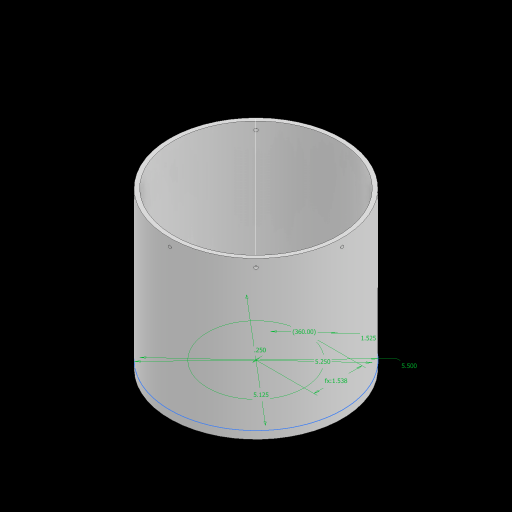
# Autodesk Inventor part: SC-1-01-Housing for Ice Holder
Saved by Autodesk Inventor 2023 (Build 270158000, 158)
## iProperties
Created: 2023-12-31
Part Number: SC-1-01-Housing for Ice Holder
Material: Generic
Document SubType Name: Modeling
Designer: annah
Density: 1 g/cm^3
Appearance: Default
Author: annah
Autodesk Inventor part; units mm, degrees
ref_plane "YZ Plane" through (0, 0, 0) normal (1, 0, 0) x (0, 1, 0)
ref_plane "XZ Plane" through (0, 0, 0) normal (0, 1, 0) x (-1, 0, 0)
sketch "Sketch1" plane through (0, 0, 0) normal (0, 1, 0) x (-1, 0, 0)
  circle A0 centre (0, 0) radius 66.675
  circle A1 centre (0, 0) radius 65.0875
  circle A2 centre (0, -39.0525) radius 19.3675
  circle A3 centre (39.0525, 0) radius 19.3675
  circle A4 centre (0, 39.0525) radius 19.3675
  circle A5 centre (-39.0525, 0) radius 19.3675
  circle A6 centre (0, 0) radius 3.175
  circle A7 centre (0, 0) radius 69.85
  dimension "d0" = 133.35
  dimension "d3" = 130.175
  dimension "d4" = 38.735
  dimension "d5" = 39.0525
  dimension "d6" = 360
  dimension "d7" = 6.35
  dimension "d8" = 139.7
  constraints: 8 centre point, 3 coincident, 9 other
  measures "d0" diameter of A0
  measures "d3" diameter of A1
  measures "d4" diameter of A2
  measures "d5" distance of point (0, 0) A2.centre
  measures "d7" diameter of A6
  measures "d8" diameter of A7
extrude "Extrusion1" add sketch "Sketch1" along normal blind 120.65 contours A7
extrude "Extrusion2" add sketch "Sketch1" against normal blind 6.35 contours A0 | A1 | A2 | A3 | A4 | A5 | A6 | A7
ref_plane "Work Plane1" through (0, 0, 69.85) normal (0, 0, 1) x (1, 0, 0)
sketch "Sketch2" plane through (0, 0, 69.85) normal (0, 0, 1) x (1, 0, 0)
  circle A0 centre (0, 114.3) radius 1.27
  line L0 (69.85, 120.65) -> (-69.85, 120.65) projected
  point P0 (0, 0)
  dimension "d14" = 2.54
  dimension "d15" = 6.35
  constraints: 1 centre point
  measures "d14" diameter of A0
  measures "d15" distance from line of L0 A0.centre
extrude "Extrusion3" cut sketch "Sketch2" against normal up to surface round surface about axis through (0, 0, 0) along (0, 1, 0) radius 66.675 far side no
pattern_circular "Circular Pattern1" count 8 over 360 about axis through (0, -10, 0) along (0, 1, 0) of "Extrusion3"
extrude "Extrusion4" add sketch "Sketch2" against normal up to surface round surface about axis through (0, 0, 0) along (0, 1, 0) radius 66.675 far side no
pattern_circular "Circular Pattern2" count 4 over 360 about axis through (0, -10, 0) along (0, 1, 0) of "Extrusion4"
sketch "Sketch3" plane through (0, -6.35, 0) normal (0, -1, 0) x (1, 0, 0)
  circle A0 centre (0, 38.1) radius 1.27
  point P0 (0, 0)
  dimension "d26" = 2.54
  dimension "d27" = 38.1
  constraints: 1 centre point
  measures "d26" diameter of A0
  measures "d27" distance of point (0, 0) A0.centre
extrude "Extrusion5" cut sketch "Sketch3" against normal up to surface (6.35 mm away)
pattern_circular "Circular Pattern3" count 4 over 360 about axis through (0, -10, 0) along (0, 1, 0) of "Extrusion5"
equation "\"d5\" = 0.3 * d3"
body "Solid1"
